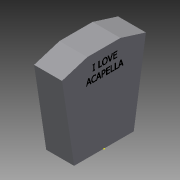
# Autodesk Inventor part: DMJ_torso
Saved by Autodesk Inventor 2015 SP1 (Build 190203100, 203)
## iProperties
Created: 2016-02-03
Part Number: DMJ_torso
Material: Generic
Document SubType Name: Modeling
Designer: guillemd
Density: 0.696303 g/cm^3
Appearance: Default
Mass: 54431.1 g
Surface Area: 11791.5 cm^2
Volume: 78171.5 cm^3
Author: guillemd
Autodesk Inventor part; units mm, degrees
ref_plane "YZ Plane" through (0, 0, 0) normal (1, 0, 0) x (0, 1, 0)
ref_plane "XZ Plane" through (0, 0, 0) normal (0, 1, 0) x (-1, 0, 0)
ref_plane "XY Plane" through (0, 0, 0) normal (0, 0, 1) x (1, 0, 0)
sketch "Sketch1" plane through (0, 0, 0) normal (1, 0, 0) x (0, 1, 0)
  line L0 (0, 190.5) -> (0, -190.5)
  line L1 (0, -190.5) -> (508, -267.97)
  line L2 (508, 267.97) -> (0, 190.5)
  line L3 (508, -267.97) -> (558.8, -105.549)
  line L4 (508, 267.97) -> (558.8, 105.549)
  line L5 (558.8, 105.549) -> (558.8, -105.549)
  point P0 (0, 0)
  point P1 (558.8, 0)
  point P2 (0, 0)
  dimension "d4" = 170.18
  dimension "d5" = 170.18
  dimension "d6" = 381
  dimension "d7" = 558.8
  dimension "d8" = 508
  dimension "d9" = 535.94
  constraints: 12 end point, 2 coincident, 2 midpoint, 2 vertical, 1 equal length, 1 horizontal alignment
  measures "d4" distance of L1.end L3.end
  measures "d5" distance of L2.start L4.end
  measures "d6" distance of L0.start L0.end
  measures "d7" distance between parallel lines of L0 L5
  measures "d8" horizontal distance of L0.end L1.end
  measures "d9" distance of L1.end L2.start
extrude "Extrusion1" add sketch "Sketch1" along normal mid plane 177.8
sketch "Sketch2" plane through (88.9, 0, 0) normal (1, 0, 0) x (0, 0, -1)
  point P0 (0, 0)
sketch "Sketch3" plane through (88.9, 0, 0) normal (1, 0, 0) x (0, 0, -1)
  line L0 (-112.634, 500.5851) -> (124.0244, 500.5851) construction
  line L1 (124.0244, 500.5851) -> (124.0244, 398.2724) construction
  line L2 (124.0244, 398.2724) -> (-112.634, 398.2724) construction
  line L3 (-112.634, 398.2724) -> (-112.634, 500.5851) construction
  point P0 (0, 0)
  constraints: 2 other
body "Solid1"
